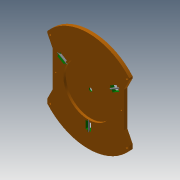
# Autodesk Inventor part: deska-pod_otocny kruh
Saved by Autodesk Inventor 2013 (Build 170138000, 138)
## iProperties
Created: 2012-09-03
Part Number: deska-pod_otocny kruh
Material: Generic
Document SubType Name: Modeling
Designer: idle-rug
Density: 1 g/cm^3
Author: idle-rug
Autodesk Inventor part; units mm, degrees
ref_plane "YZ Plane" through (0, 0, 0) normal (1, 0, 0) x (0, 1, 0)
ref_plane "XZ Plane" through (0, 0, 0) normal (0, 1, 0) x (-1, 0, 0)
ref_plane "XY Plane" through (0, 0, 0) normal (0, 0, 1) x (1, 0, 0)
sketch "Sketch1" plane through (0, 0, 0) normal (0, 1, 0) x (-1, 0, 0)
  circle A0 centre (24.1, 110.65) radius 0.25
  circle A1 centre (-70.5, 110.65) radius 0.25
  circle A2 centre (-45.6, 89.15) radius 0.25
  circle A3 centre (0, 67.65) radius 0.25
  circle A4 centre (70.5, 42.15) radius 0.25
  circle A5 centre (32.15, 17.15) radius 0.25
  circle A6 centre (60.5, -17.65) radius 0.25
  circle A7 centre (-60.5, -17.65) radius 0.25
  circle A8 centre (24.1, -67.65) radius 0.25
  circle A9 centre (-70.5, -67.65) radius 0.25
  circle A10 centre (-45.6, -89.15) radius 0.25
  circle A11 centre (0, -110.65) radius 0.25
  circle A12 centre (-70.5, -110.65) radius 0.25
  circle A13 centre (70.5, -110.65) radius 0.25
  circle A14 centre (45.6, -89.15) radius 0.25
  circle A15 centre (-24.1, -67.65) radius 0.25
  circle A16 centre (70.5, -67.65) radius 0.25
  circle A17 centre (0, -17.65) radius 0.25
  circle A18 centre (-32.15, 17.15) radius 0.25
  circle A19 centre (-70.5, 42.15) radius 0.25
  circle A20 centre (-70.5, 67.65) radius 0.25
  circle A21 centre (70.5, 67.65) radius 0.25
  circle A22 centre (45.6, 89.15) radius 0.25
  circle A23 centre (-24.1, 110.65) radius 0.25
  circle A24 centre (70.5, 110.65) radius 0.25
  line L0 (75.5, -115.65) -> (75.5, -62.65)
  line L1 (75.5, -62.65) -> (65.5, -42.65)
  line L2 (65.5, -42.65) -> (65.5, 22.15)
  line L3 (65.5, 22.15) -> (75.5, 42.15)
  line L4 (75.5, 42.15) -> (75.5, 115.65)
  line L5 (75.5, 115.65) -> (30.5, 135.65)
  line L6 (30.5, 135.65) -> (-30.5, 135.65)
  line L7 (-30.5, 135.65) -> (-75.5, 115.65)
  line L8 (-75.5, 115.65) -> (-75.5, 42.15)
  line L9 (-75.5, 42.15) -> (-65.5, 22.15)
  line L10 (-65.5, 22.15) -> (-65.5, -42.65)
  line L11 (-65.5, -42.65) -> (-75.5, -62.65)
  line L12 (-75.5, -62.65) -> (-75.5, -115.65)
  line L13 (-75.5, -115.65) -> (-30.5, -135.65)
  line L14 (-30.5, -135.65) -> (30.5, -135.65)
  line L15 (30.5, -135.65) -> (75.5, -115.65)
  circle A25 centre (0, -110.65) radius 2
  circle A26 centre (70.5, -110.65) radius 2
  circle A27 centre (-70.5, -110.65) radius 2
  circle A28 centre (45.6, -89.15) radius 2
  circle A29 centre (-45.6, -89.15) radius 2
  circle A30 centre (70.5, -67.65) radius 2
  circle A31 centre (24.1, -67.65) radius 2
  circle A32 centre (-24.1, -67.65) radius 2
  circle A33 centre (-70.5, -67.65) radius 2
  circle A34 centre (60.5, -17.65) radius 2
  circle A35 centre (0, -17.65) radius 2
  circle A36 centre (-32.15, 17.15) radius 2
  circle A37 centre (-60.5, -17.65) radius 2
  circle A38 centre (32.15, 17.15) radius 2
  circle A39 centre (70.5, 42.15) radius 2
  circle A40 centre (-70.5, 42.15) radius 2
  circle A41 centre (-70.5, 67.65) radius 2
  circle A42 centre (0, 67.65) radius 2
  circle A43 centre (70.5, 67.65) radius 2
  circle A44 centre (45.6, 89.15) radius 2
  circle A45 centre (-45.6, 89.15) radius 2
  circle A46 centre (-70.5, 110.65) radius 2
  circle A47 centre (-24.1, 110.65) radius 2
  circle A48 centre (24.1, 110.65) radius 2
  circle A49 centre (70.5, 110.65) radius 2
  point P0 (0, 0)
  point P1 (0, 0)
  dimension "d0" = 4
  dimension "d1" = 4
  dimension "d2" = 4
  dimension "d3" = 4
  dimension "d4" = 4
  dimension "d5" = 4
  dimension "d6" = 4
  dimension "d7" = 4
  dimension "d8" = 4
  dimension "d9" = 4
  dimension "d10" = 4
  dimension "d11" = 4
  dimension "d12" = 4
  dimension "d13" = 4
  dimension "d14" = 4
  dimension "d15" = 4
  dimension "d16" = 4
  dimension "d17" = 4
  dimension "d18" = 4
  dimension "d19" = 4
  dimension "d20" = 4
  dimension "d21" = 4
  dimension "d22" = 4
  dimension "d23" = 4
  dimension "d24" = 4
  constraints: 50 centre point, 32 end point, 25 coincident
  measures "d0" diameter of A25
  measures "d1" diameter of A26
  measures "d2" diameter of A27
  measures "d3" diameter of A28
  measures "d4" diameter of A29
  measures "d5" diameter of A30
  measures "d6" diameter of A31
  measures "d7" diameter of A32
  measures "d8" diameter of A33
  measures "d9" diameter of A34
  measures "d10" diameter of A35
  measures "d11" diameter of A36
  measures "d12" diameter of A37
  measures "d13" diameter of A38
  measures "d14" diameter of A39
  measures "d15" diameter of A40
  measures "d16" diameter of A41
  measures "d17" diameter of A42
  measures "d18" diameter of A43
  measures "d19" diameter of A44
  measures "d20" diameter of A45
  measures "d21" diameter of A46
  measures "d22" diameter of A47
  measures "d23" diameter of A48
  measures "d24" diameter of A49
extrude "Extrusion1" add sketch "Sketch1" along normal blind 2 contours L15 L14 L13 L12 L11 L10 L9 L8 L7 L6 L5 L4 L3 L2 L1 L0
sketch "Sketch2" plane through (0, 0, 0) normal (0, -1, 0) x (1, 0, 0)
  circle A0 centre (-70.5, 110.65) radius 2 projected
  circle A1 centre (-24.1, 110.65) radius 2 projected
  circle A2 centre (24.1, 110.65) radius 2 projected
  circle A3 centre (70.5, 110.65) radius 2 projected
  circle A4 centre (45.6, 89.15) radius 2 projected
  circle A5 centre (-45.6, 89.15) radius 2 projected
  circle A6 centre (-70.5, 67.65) radius 2 projected
  circle A7 centre (0, 67.65) radius 2 projected
  circle A8 centre (70.5, 67.65) radius 2 projected
  circle A9 centre (70.5, 42.15) radius 2 projected
  circle A10 centre (-70.5, 42.15) radius 2 projected
  circle A11 centre (-32.15, 17.15) radius 2 projected
  circle A12 centre (60.5, -17.65) radius 2 projected
  circle A13 centre (32.15, 17.15) radius 2 projected
  circle A14 centre (0, -17.65) radius 2 projected
  circle A15 centre (-60.5, -17.65) radius 2 projected
  circle A16 centre (70.5, -67.65) radius 2 projected
  circle A17 centre (24.1, -67.65) radius 2 projected
  circle A18 centre (-24.1, -67.65) radius 2 projected
  circle A19 centre (-70.5, -67.65) radius 2 projected
  circle A20 centre (45.6, -89.15) radius 2 projected
  circle A21 centre (-45.6, -89.15) radius 2 projected
  circle A22 centre (70.5, -110.65) radius 2 projected
  circle A23 centre (-70.5, -110.65) radius 2 projected
  circle A24 centre (0, -110.65) radius 2 projected
  line L0 (65.5, 22.15) -> (75.5, 42.15) projected
  line L1 (75.5, 42.15) -> (75.5, 115.65) projected
  line L2 (75.5, 115.65) -> (30.5, 135.65) projected
  line L3 (30.5, 135.65) -> (-30.5, 135.65) projected
  line L4 (-30.5, 135.65) -> (-75.5, 115.65) projected
  line L5 (-75.5, 115.65) -> (-75.5, 42.15) projected
  line L6 (-75.5, 42.15) -> (-65.5, 22.15) projected
  line L7 (-65.5, 22.15) -> (-65.5, -42.65) projected
  line L8 (-65.5, -42.65) -> (-75.5, -62.65) projected
  line L9 (-75.5, -62.65) -> (-75.5, -115.65) projected
  line L10 (-75.5, -115.65) -> (-30.5, -135.65) projected
  line L11 (-30.5, -135.65) -> (30.5, -135.65) projected
  line L12 (30.5, -135.65) -> (75.5, -115.65) projected
  line L13 (75.5, -115.65) -> (75.5, -62.65) projected
  line L14 (75.5, -62.65) -> (65.5, -42.65) projected
  line L15 (65.5, -42.65) -> (65.5, 22.15) projected
  point P0 (0, 0)
extrude "Extrusion2" add sketch "Sketch2" along normal blind 1.3
sketch "Sketch3" plane through (0, -1.3, 0) normal (0, -1, 0) x (1, 0, 0)
  circle A0 centre (0, -110.65) radius 2 projected
  circle A1 centre (-70.5, -110.65) radius 2 projected
  circle A2 centre (70.5, -110.65) radius 2 projected
  circle A3 centre (-45.6, -89.15) radius 2 projected
  circle A4 centre (45.6, -89.15) radius 2 projected
  circle A5 centre (-70.5, -67.65) radius 2 projected
  circle A6 centre (-24.1, -67.65) radius 2 projected
  circle A7 centre (24.1, -67.65) radius 2 projected
  circle A8 centre (70.5, -67.65) radius 2 projected
  circle A9 centre (-60.5, -17.65) radius 2 projected
  circle A10 centre (0, -17.65) radius 2 projected
  circle A11 centre (32.15, 17.15) radius 2 projected
  circle A12 centre (60.5, -17.65) radius 2 projected
  circle A13 centre (-32.15, 17.15) radius 2 projected
  circle A14 centre (-70.5, 42.15) radius 2 projected
  circle A15 centre (70.5, 42.15) radius 2 projected
  circle A16 centre (70.5, 67.65) radius 2 projected
  circle A17 centre (0, 67.65) radius 2 projected
  circle A18 centre (-70.5, 67.65) radius 2 projected
  circle A19 centre (-45.6, 89.15) radius 2 projected
  circle A20 centre (45.6, 89.15) radius 2 projected
  circle A21 centre (70.5, 110.65) radius 2 projected
  circle A22 centre (24.1, 110.65) radius 2 projected
  circle A23 centre (-24.1, 110.65) radius 2 projected
  circle A24 centre (-70.5, 110.65) radius 2 projected
  line L0 (65.5, 22.15) -> (75.5, 42.15) projected
  line L1 (75.5, 42.15) -> (75.5, 115.65) projected
  line L2 (75.5, 115.65) -> (30.5, 135.65) projected
  line L3 (30.5, 135.65) -> (-30.5, 135.65) projected
  line L4 (-30.5, 135.65) -> (-75.5, 115.65) projected
  line L5 (-75.5, 115.65) -> (-75.5, 42.15) projected
  line L6 (-75.5, 42.15) -> (-65.5, 22.15) projected
  line L7 (-65.5, 22.15) -> (-65.5, -42.65) projected
  line L8 (-65.5, -42.65) -> (-75.5, -62.65) projected
  line L9 (-75.5, -62.65) -> (-75.5, -115.65) projected
  line L10 (-75.5, -115.65) -> (-30.5, -135.65) projected
  line L11 (-30.5, -135.65) -> (30.5, -135.65) projected
  line L12 (30.5, -135.65) -> (75.5, -115.65) projected
  line L13 (75.5, -115.65) -> (75.5, -62.65) projected
  line L14 (75.5, -62.65) -> (65.5, -42.65) projected
  line L15 (65.5, -42.65) -> (65.5, 22.15) projected
  point P0 (0, 0)
extrude "Extrusion3" add sketch "Sketch3" along normal blind 8
sketch "Sketch4" plane through (0, 2, 0) normal (0, 1, 0) x (1, 0, 0)
  circle A0 centre (-32.15, -17.15) radius 2 projected
  circle A1 centre (60.5, 17.65) radius 2 projected
  circle A2 centre (32.15, -17.15) radius 2 projected
  circle A3 centre (0, 17.65) radius 2 projected
  circle A4 centre (-60.5, 17.65) radius 2 projected
  point P0 (0, 0)
extrude "Extrusion4" add sketch "Sketch4" against normal blind 10
sketch "Sketch5" plane through (0, 2, 0) normal (0, 1, 0) x (1, 0, 0)
  circle A0 centre (-70.5, -67.65) radius 2 projected
  circle A1 centre (0, -67.65) radius 2 projected
  circle A2 centre (70.5, -67.65) radius 2 projected
  circle A3 centre (24.1, 67.65) radius 2 projected
  circle A4 centre (-24.1, 67.65) radius 2 projected
  point P0 (0, 0)
extrude "Extrusion5" add sketch "Sketch5" against normal blind 10
sketch "Sketch6" plane through (0, -9.3, 0) normal (0, -1, 0) x (1, 0, 0)
  line L0 (75.5, 115.65) -> (30.5, 135.65) projected
  line L1 (30.5, 135.65) -> (-30.5, 135.65) projected
  line L2 (-30.5, 135.65) -> (-75.5, 115.65) projected
  line L3 (-75.5, -115.65) -> (-30.5, -135.65) projected
  line L4 (-30.5, -135.65) -> (30.5, -135.65) projected
  line L5 (30.5, -135.65) -> (75.5, -115.65) projected
  line L6 (-75.5, 42.15) -> (-75.5, 45.15)
  line L7 (-75.5, 45.15) -> (75.5, 45.15)
  line L8 (75.5, 45.15) -> (75.5, 42.15)
  line L9 (-75.5, -62.65) -> (-75.5, -70.65)
  line L10 (-75.5, -115.65) -> (-75.5, -62.65) projected
  line L11 (-75.5, -70.65) -> (75.5, -70.65)
  line L12 (75.5, -70.65) -> (75.5, -62.65)
  line L13 (-75.5, -70.65) -> (-75.5, -115.65)
  line L14 (-75.5, -62.65) -> (-75.5, -115.65) projected
  line L15 (75.5, -70.65) -> (75.5, -115.65)
  line L16 (75.5, 45.15) -> (75.5, 115.65)
  line L17 (-75.5, 115.65) -> (-75.5, 45.15)
  point P0 (0, 0)
  dimension "d35" = 3
  dimension "d36" = 8
  constraints: 20 end point, 2 collinear, 2 parallel, 1 perpendicular, 1 point on line
  measures "d35" distance of L6.start L6.end
  measures "d36" distance of L9.start L9.end
extrude "Extrusion6" cut sketch "Sketch6" against normal blind 11.3
sketch "Sketch7" plane through (0, -9.3, 0) normal (0, -1, 0) x (1, 0, 0)
  circle A0 centre (-32.15, 17.15) radius 2 projected
  circle A1 centre (32.15, 17.15) radius 2 projected
  circle A2 centre (0, -17.65) radius 2 projected
  circle A3 centre (24.1, -67.65) radius 2 projected
  circle A4 centre (-24.1, -67.65) radius 2 projected
  point P0 (0, 0)
extrude "Extrusion7" add sketch "Sketch7" against normal blind 11.3
sketch "Sketch9" plane through (-60.5, -8, -17.65) normal (0, -1, 0) x (1, 0, 0)
  circle A0 centre (0, 0) radius 2 projected
  point P0 (60.5, 17.65)
sketch "Sketch10" plane through (60.5, -8, -17.65) normal (0, -1, 0) x (1, 0, 0)
  circle A0 centre (0, 0) radius 2 projected
  point P0 (-60.5, 17.65)
extrude "Extrusion8" cut sketch "Sketch9" against normal blind 11.3
extrude "Extrusion9" cut sketch "Sketch10" against normal blind 11.3
sketch "Sketch11" plane through (0, -9.3, 0) normal (0, -1, 0) x (1, 0, 0)
  line L0 (-75.5, -70.65) -> (75.5, -70.65)
  line L1 (75.5, 45.15) -> (-75.5, 45.15)
  arc A0 (75.5, 45.15) -> (-75.5, 45.15) centre (0, -20.422479) ccw
  arc A1 (-75.5, -70.65) -> (75.5, -70.65) centre (0, -5.077521) ccw
  point P0 (0, 0)
  dimension "d45" = 100
  dimension "d46" = 100
  constraints: 4 point on circle, 2 centre point
  measures "d45" radius of A0
  measures "d46" radius of A1
extrude "Extrusion10" add sketch "Sketch11" against normal blind 11.3
sketch "Sketch12" plane through (0, -9.3, 0) normal (0, -1, 0) x (1, 0, 0)
  arc A0 (75.5, 45.15) -> (-75.5, 45.15) centre (0, -20.422479) ccw
  arc A1 (-75.5, -70.65) -> (75.5, -70.65) centre (0, -5.077521) ccw
  line L0 (0, 79.577521) -> (0, -105.077521)
  circle A2 centre (0, -12.75) radius 3
  point P0 (0, 0)
  dimension "d49" = 6
  constraints: 2 end point, 2 point on circle, 1 centre point, 1 midpoint
  measures "d49" diameter of A2
extrude "Extrusion11" cut sketch "Sketch12" against normal blind 11.3
sketch "Sketch13" plane through (0, -9.3, 0) normal (0, -1, 0) x (1, 0, 0)
  line L0 (-65.5, -42.65) -> (-65.5, 22.15) projected
  circle A0 centre (-60.5, -12.75) radius 1.5
  circle A1 centre (60.5, -12.75) radius 1.5
  point P0 (0, 0)
  dimension "d52" = 3
  dimension "d53" = 3
  constraints: 2 centre point
  measures "d52" diameter of A0
  measures "d53" diameter of A1
extrude "Extrusion12" cut sketch "Sketch13" against normal blind 11.3
sketch "Sketch14" plane through (0, -9.3, 0) normal (0, -1, 0) x (1, 0, 0)
  circle A0 centre (60.5, -17.65) radius 2 projected
  circle A1 centre (-60.5, -17.65) radius 2 projected
  point P0 (0, 0)
extrude "Extrusion13" add sketch "Sketch14" against normal blind 11.3
sketch "Sketch15" plane through (0, -9.3, 0) normal (0, -1, 0) x (1, 0, 0)
  circle A0 centre (-60.5, -12.75) radius 1.5
  circle A1 centre (60.5, -12.75) radius 1.5
  circle A2 centre (0, -12.75) radius 3
  line L0 (75.5, -70.65) -> (75.5, -62.65)
  line L1 (75.5, -62.65) -> (65.5, -42.65)
  line L2 (65.5, -42.65) -> (65.5, 22.15)
  line L3 (65.5, 22.15) -> (75.5, 42.15)
  line L4 (75.5, 42.15) -> (75.5, 45.15)
  arc A3 (75.5, 45.15) -> (-75.5, 45.15) centre (0, -20.422479) ccw
  line L5 (-75.5, 45.15) -> (-75.5, 42.15)
  line L6 (-75.5, 42.15) -> (-65.5, 22.15)
  line L7 (-65.5, 22.15) -> (-65.5, -42.65)
  line L8 (-65.5, -42.65) -> (-75.5, -62.65)
  line L9 (-75.5, -62.65) -> (-75.5, -70.65)
  arc A4 (-75.5, -70.65) -> (75.5, -70.65) centre (0, -5.077521) ccw
  circle A5 centre (70.5, 42.15) radius 2
  circle A6 centre (-70.5, 42.15) radius 2
  circle A7 centre (70.5, -67.65) radius 2
  circle A8 centre (-70.5, -67.65) radius 2
  point P0 (0, 0)
extrude "Extrusion14" cut sketch "Sketch15" against normal blind 1.3
sketch "Sketch16" plane through (0, -8, 0) normal (0, -1, 0) x (1, 0, 0)
  circle A0 centre (0, -12.75) radius 3 projected
  circle A1 centre (0, -12.75) radius 60
  circle A2 centre (0, -12.75) radius 30.0955
  line L0 (0, -12.75) -> (0, -49.95)
  circle A3 centre (0, -49.95) radius 7.1045
  circle A4 centre (0, -12.75) radius 45.75
  point P0 (0, 0)
  dimension "d60" = 120
  dimension "d63" = 60.191
  dimension "d65" = 37.2
  dimension "d66" = 14.209
  dimension "d67" = 91.5
  constraints: 4 centre point, 4 coincident, 2 end point
  measures "d60" diameter of A1
  measures "d63" diameter of A2
  measures "d65" distance of L0.start L0.end
  measures "d66" diameter of A3
  measures "d67" diameter of A4
extrude "Extrusion15" cut sketch "Sketch16" against normal blind 8 contours A2 | A3 | A4
sketch "Sketch17" plane through (0, -8, 0) normal (0, -1, 0) x (1, 0, 0)
  circle A0 centre (0, -12.75) radius 45.75
  circle A1 centre (-70.5, -67.65) radius 2
  circle A2 centre (70.5, -67.65) radius 2
  circle A3 centre (-70.5, 42.15) radius 2
  circle A4 centre (70.5, 42.15) radius 2
  circle A5 centre (60.5, -12.75) radius 1.5
  circle A6 centre (-60.5, -12.75) radius 1.5
  line L0 (75.5, -62.65) -> (75.5, -70.65)
  line L1 (65.5, -42.65) -> (75.5, -62.65)
  line L2 (65.5, 22.15) -> (65.5, -42.65)
  line L3 (75.5, 42.15) -> (65.5, 22.15)
  line L4 (75.5, 45.15) -> (75.5, 42.15)
  arc A7 (75.5, 45.15) -> (-75.5, 45.15) centre (0, -20.422479) ccw
  line L5 (-75.5, 42.15) -> (-75.5, 45.15)
  line L6 (-65.5, 22.15) -> (-75.5, 42.15)
  line L7 (-65.5, -42.65) -> (-65.5, 22.15)
  line L8 (-75.5, -62.65) -> (-65.5, -42.65)
  line L9 (-75.5, -70.65) -> (-75.5, -62.65)
  arc A8 (-75.5, -70.65) -> (75.5, -70.65) centre (0, -5.077521) ccw
  point P0 (0, 0)
extrude "Extrusion16" cut sketch "Sketch17" against normal blind 3.8
sketch "Sketch18" plane through (0, -4.2, 0) normal (0, -1, 0) x (1, 0, 0)
  circle A0 centre (0, -12.75) radius 45.75
  line L0 (5, -58.5) -> (-5, -58.5)
  line L1 (-5, -58.5) -> (-5, -78.5)
  line L2 (-5, -78.5) -> (5, -78.5)
  line L3 (5, -78.5) -> (5, -58.5)
  circle A1 centre (0, -12.75) radius 3
  arc A2 (-75.5, -70.65) -> (75.5, -70.65) centre (0, -5.077521) ccw
  line L4 (5, -75.5) -> (-5, -75.5)
  line L5 (-5, -75.5) -> (-5, -61.5)
  line L6 (-5, -61.5) -> (5, -61.5)
  line L7 (5, -61.5) -> (5, -75.5)
  line L8 (5, -75.5) -> (-5, -61.5) construction
  line L9 (-5, -75.5) -> (5, -61.5) construction
  line L10 (0, -12.75) -> (89.8, -12.75) construction
  line L11 (0, -12.75) -> (60, -12.75) construction
  line L12 (0, -12.75) -> (60, -12.75) construction
  line L13 (0, -12.75) -> (60, -12.75) construction
  circle A3 centre (0, -12.75) radius 3
  line L14 (-59.44117, 15.794873) -> (-42.120662, 5.794873)
  line L15 (-42.120662, 5.794873) -> (-37.120662, 14.455127)
  line L16 (-37.120662, 14.455127) -> (-54.44117, 24.455127)
  line L17 (-54.44117, 24.455127) -> (-59.44117, 15.794873)
  line L18 (-59.44117, 15.794873) -> (-37.120662, 14.455127) construction
  line L19 (-42.120662, 5.794873) -> (-54.44117, 24.455127) construction
  line L20 (59.44117, 15.794873) -> (42.120662, 5.794873)
  line L21 (42.120662, 5.794873) -> (37.120662, 14.455127)
  line L22 (37.120662, 14.455127) -> (54.44117, 24.455127)
  line L23 (54.44117, 24.455127) -> (59.44117, 15.794873)
  line L24 (59.44117, 15.794873) -> (37.120662, 14.455127) construction
  line L25 (42.120662, 5.794873) -> (54.44117, 24.455127) construction
  line L26 (-51.843094, 22.955127) -> (-39.718738, 15.955127)
  line L27 (-39.718738, 15.955127) -> (-44.718738, 7.294873)
  line L28 (-44.718738, 7.294873) -> (-56.843094, 14.294873)
  line L29 (-56.843094, 14.294873) -> (-51.843094, 22.955127)
  line L30 (-51.843094, 22.955127) -> (-44.718738, 7.294873) construction
  line L31 (-39.718738, 15.955127) -> (-56.843094, 14.294873) construction
  line L32 (56.843094, 14.294873) -> (44.718738, 7.294873)
  line L33 (44.718738, 7.294873) -> (39.718738, 15.955127)
  line L34 (39.718738, 15.955127) -> (51.843094, 22.955127)
  line L35 (51.843094, 22.955127) -> (56.843094, 14.294873)
  line L36 (56.843094, 14.294873) -> (39.718738, 15.955127) construction
  line L37 (44.718738, 7.294873) -> (51.843094, 22.955127) construction
  line L38 (-42.218738, 11.625) -> (-39.620662, 10.125)
  circle A4 centre (0, -12.75) radius 45.75
  line L39 (-42.218738, 11.625) -> (-39.218738, 11.625) construction
  line L40 (42.218738, 11.625) -> (39.620662, 10.125)
  line L41 (0, -61.5) -> (0, -58.5)
  line L42 (0, -75.5) -> (0, -78.5)
  line L43 (-56.94117, 20.125) -> (-54.343094, 18.625)
  line L44 (56.94117, 20.125) -> (54.343094, 18.625)
  line L45 (-41.593738, 12.707532) -> (-38.995662, 11.207532)
  line L46 (-38.995662, 11.207532) -> (-40.245662, 9.042468)
  line L47 (-40.245662, 9.042468) -> (-42.843738, 10.542468)
  line L48 (-42.843738, 10.542468) -> (-41.593738, 12.707532)
  line L49 (-41.593738, 12.707532) -> (-40.245662, 9.042468) construction
  line L50 (-38.995662, 11.207532) -> (-42.843738, 10.542468) construction
  line L51 (-53.718094, 19.707532) -> (-56.31617, 21.207532)
  line L52 (-56.31617, 21.207532) -> (-57.56617, 19.042468)
  line L53 (-57.56617, 19.042468) -> (-54.968094, 17.542468)
  line L54 (-54.968094, 17.542468) -> (-53.718094, 19.707532)
  line L55 (-53.718094, 19.707532) -> (-57.56617, 19.042468) construction
  line L56 (-56.31617, 21.207532) -> (-54.968094, 17.542468) construction
  line L57 (42.843738, 10.542468) -> (40.245662, 9.042468)
  line L58 (40.245662, 9.042468) -> (38.995662, 11.207532)
  line L59 (38.995662, 11.207532) -> (41.593738, 12.707532)
  line L60 (41.593738, 12.707532) -> (42.843738, 10.542468)
  line L61 (42.843738, 10.542468) -> (38.995662, 11.207532) construction
  line L62 (40.245662, 9.042468) -> (41.593738, 12.707532) construction
  line L63 (57.56617, 19.042468) -> (54.968094, 17.542468)
  line L64 (54.968094, 17.542468) -> (53.718094, 19.707532)
  line L65 (53.718094, 19.707532) -> (56.31617, 21.207532)
  line L66 (56.31617, 21.207532) -> (57.56617, 19.042468)
  line L67 (57.56617, 19.042468) -> (53.718094, 19.707532) construction
  line L68 (54.968094, 17.542468) -> (56.31617, 21.207532) construction
  line L69 (1.25, -58.5) -> (1.25, -61.5)
  line L70 (1.25, -61.5) -> (-1.25, -61.5)
  line L71 (-1.25, -61.5) -> (-1.25, -58.5)
  line L72 (-1.25, -58.5) -> (1.25, -58.5)
  line L73 (1.25, -58.5) -> (-1.25, -61.5) construction
  line L74 (1.25, -61.5) -> (-1.25, -58.5) construction
  line L75 (1.25, -75.5) -> (1.25, -78.5)
  line L76 (1.25, -78.5) -> (-1.25, -78.5)
  line L77 (-1.25, -78.5) -> (-1.25, -75.5)
  line L78 (-1.25, -75.5) -> (1.25, -75.5)
  line L79 (1.25, -75.5) -> (-1.25, -78.5) construction
  line L80 (1.25, -78.5) -> (-1.25, -75.5) construction
  point P0 (0, 0)
  point P1 (-40.9197, 10.875)
  point P2 (-55.642132, 19.375)
  point P3 (40.9197, 10.875)
  point P4 (55.642132, 19.375)
  point P5 (0, -60)
  point P6 (0, -77)
  dimension "d72" = 10
  dimension "d73" = 20
  dimension "d74" = 10
  dimension "d75" = 14
  dimension "d87" = 20
  dimension "d88" = 10
  dimension "d89" = 20
  dimension "d90" = 10
  dimension "d91" = 14
  dimension "d92" = 10
  dimension "d93" = 14
  dimension "d94" = 10
  dimension "d97" = 30
  dimension "d98" = 2.5
  dimension "d99" = 2.5
  dimension "d100" = 2.5
  dimension "d101" = 2.5
  dimension "d102" = 2.5
  dimension "d103" = 2.5
  constraints: 162 end point, 31 equal length, 29 midpoint, 13 perpendicular, 7 horizontal, 2 point on circle, 1 coincident, 1 vertical alignment, 1 other
  measures "d72" distance of L2.end L1.end
  measures "d73" distance of L1.end L0.end
  measures "d74" distance of L5.end L6.end
  measures "d75" distance of L4.end L5.end
  measures "d87" distance of L14.start L14.end
  measures "d88" distance of L15.end L14.end
  measures "d89" distance of L20.start L20.end
  measures "d90" distance of L20.end L21.end
  measures "d91" distance of L26.start L26.end
  measures "d92" distance of L26.end L27.end
  measures "d93" distance of L32.start L32.end
  measures "d94" distance of L32.end L33.end
  measures "d97" angle of L38 L39
  measures "d98" distance of L45.end L46.end
  measures "d99" distance of L52.end L51.end
  measures "d100" distance of L57.end L58.end
  measures "d101" distance of L63.end L64.end
  measures "d102" distance of L69.end L70.end
  measures "d103" distance of L75.end L76.end
extrude "Extrusion17" cut sketch "Sketch18" against normal blind 10 contours L33 L22 L35 L20 | L6 L3 L4 L1 | L27 L14 L29 L16
extrude "Extrusion18" cut sketch "Sketch18" against normal blind 2.5 contours L0 L69 L6 L41 | L41 L6 L71 L0 | L15 L47 L27 L38 | L38 L27 L45 L15 | L21 L59 L33 L40 | L40 L33 L57 L21 | L35 L44 L23 L63 | L65 L23 L44 L35 | L75 L2 L42 L4 | L4 L42 L2 L77 | L53 L17 L43 L29 | L29 L43 L17 L51
sketch "Sketch19" plane through (-57.56617, -4.2, 19.042468) normal (0.8660254, 0, -0.5) x (-0.5, 0, -0.8660254)
  circle A0 centre (-1.25, 1.25) radius 1.25
  point P0 (-12.291824, 4.2)
  constraints: 1 centre point
extrude "Extrusion19" add sketch "Sketch19" along normal blind 20
sketch "Sketch20" plane through (56.31617, -4.2, 21.207532) normal (-0.8660254, 0, -0.5) x (-0.5, 0, 0.8660254)
  circle A0 centre (-1.25, 1.25) radius 1.25
  point P0 (9.791824, 4.2)
  constraints: 1 centre point
extrude "Extrusion20" add sketch "Sketch20" along normal blind 20
sketch "Sketch21" plane through (-1.25, -4.2, -78.5) normal (0, 0, 1) x (1, 0, 0)
  circle A0 centre (1.25, 1.25) radius 1.25
  point P0 (1.25, 4.2)
  constraints: 1 centre point
extrude "Extrusion21" add sketch "Sketch21" along normal blind 20
body "Solid1"
